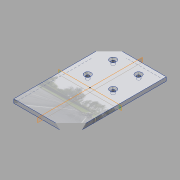
# Autodesk Inventor part: PBLMK-041-5
Saved by Autodesk Inventor 2016 (Build 200138000, 138)
## iProperties
Created: 2024-01-03
Part Number: PBLMK-041-5
Material: Generic
Document SubType Name: Modeling
Designer: Riskinova Oktavia
Density: 1 g/cm^3
Appearance: Aluminum - Flat
Description: LASER BASE
Author: Riskinova Oktavia
Autodesk Inventor part; units mm, degrees
ref_plane "XY Plane" through (0, 0, 0) normal (0, 0, 1) x (1, 0, 0)
sketch "Sketch1" plane through (0, 0, 0) normal (0, 0, 1) x (1, 0, 0)
  line L0 (-45, -65) -> (45, -65)
  line L1 (45, -65) -> (45, 65)
  line L2 (45, 65) -> (-45, 65)
  line L3 (-45, 65) -> (-45, -65)
  line L4 (-45, -65) -> (45, 65) construction
  line L5 (45, -65) -> (-45, 65) construction
  line L6 (228, -13.575) -> (-228, -13.575) projected
  point P0 (0, 0)
  dimension "d0" = 90
  dimension "d1" = 130
  constraints: 12 end point, 2 midpoint, 2 parallel, 1 horizontal, 1 perpendicular
  measures "d0" distance of L1.end L2.end
  measures "d1" distance of L0.end L1.end
extrude "Extrusion1" add sketch "Sketch1" along normal mid plane 6
sketch "Sketch2" plane through (0, 0, 3) normal (0, 0, 1) x (1, 0, 0)
  point P0 (0, 0)
sketch "Sketch3" plane through (0, 0, 3) normal (0, 0, 1) x (1, 0, 0)
  circle A0 centre (-20, 46.425) radius 2.1
  circle A1 centre (20, 46.425) radius 2.1
  circle A2 centre (-20, 6.425) radius 2.1
  circle A3 centre (20, 6.425) radius 2.1
  circle A4 centre (-20, 6.425) radius 2.1 projected
  circle A5 centre (20, 6.425) radius 2.1 projected
  circle A6 centre (-20, 46.425) radius 2.1 projected
  circle A7 centre (20, 46.425) radius 2.1 projected
  point P0 (0, 0)
  constraints: 4 centre point, 4 coincident, 4 concentric
hole "Hole1" at (-20, 46.425, 3) at (20, 46.425, 3) at (-20, 6.425, 3) at (20, 6.425, 3) direction (0, 0, -1) diameter 5.5 end through all countersink diameter 10.4 countersink angle 90 clearance for "Countersunk Flat Head Screw ISO 2009/7046" size "M5" standard "ISO"
body "Solid1"
